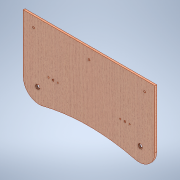
# Autodesk Inventor part: FTC Outside Panels
Saved by Autodesk Inventor 2020 (Build 240168000, 168)
## iProperties
Created: 2022-09-23
Part Number: FTC Outside Panels
Material: Wood (Oak)
Document SubType Name: Modeling
Designer: Jason
Density: 0.76 g/cm^3
Appearance: White Oak - Natural Medium Gloss
Author: Jason
Autodesk Inventor part; units mm, degrees
ref_plane "YZ Plane" through (0, 0, 0) normal (1, 0, 0) x (0, 1, 0)
ref_plane "XZ Plane" through (0, 0, 0) normal (0, 1, 0) x (-1, 0, 0)
ref_plane "XY Plane" through (0, 0, 0) normal (0, 0, 1) x (1, 0, 0)
sketch "Sketch1" plane through (0, 0, 0) normal (0, 0, 1) x (1, 0, 0)
  line L0 (49.2125, 0) -> (54.6328, 0)
  line L1 (357.1875, 0) -> (350.9902, 0)
  arc A0 (0, 49.2125) -> (65.0875, 2.6308) centre (49.2125, 49.2125) ccw
  arc A1 (345.2239, 1.4763) -> (406.4, 49.2125) centre (357.1875, 49.2125) ccw
  arc A2 (203.2, 19.05) -> (54.6328, 0) centre (202.8115, -566.7686) ccw
  arc A3 (350.9902, 0) -> (345.2239, 1.4763) centre (202.8115, -566.7686) ccw
  arc A4 (65.0875, 2.6308) -> (54.6328, 0) centre (202.8115, -566.7686) ccw
  arc A5 (350.9902, 0) -> (203.2, 19.05) centre (202.8115, -566.7686) ccw
  line L2 (0, 49.2125) -> (0, 228.6)
  line L3 (406.4, 228.6) -> (406.4, 49.2125)
  line L4 (0, 228.6) -> (406.4, 228.6)
  point P0 (0, 0)
  point P1 (57.0671, 0.6309)
  constraints: 16 point on circle, 10 end point, 6 centre point, 1 perpendicular, 1 vertical
extrude "Extrusion1" add sketch "Sketch1" along normal blind 5.5563 contours A0 L2 L4 L3 A1 A5 A2
sketch "Sketch2" plane through (0, 0, 5.5563) normal (0, 0, 1) x (1, 0, 0)
  arc A0 (0, 49.2125) -> (57.0671, 0.6309) centre (49.2125, 49.2125) ccw projected
  arc A1 (345.2239, 1.4763) -> (406.4, 49.2125) centre (357.1875, 49.2125) ccw projected
  line L0 (361.7622, 0.2131) -> (361.7412, 44.6631)
  line L1 (361.7412, 44.6631) -> (406.1912, 44.6631)
  line L2 (0.2109, 44.6609) -> (44.6609, 44.6609)
  line L3 (44.6609, 44.6609) -> (44.6609, 0.2109)
  line L4 (365.2681, 38.3131) -> (368.9342, 44.6631)
  line L5 (365.2681, 51.0131) -> (368.9342, 44.6631)
  line L6 (357.9357, 51.0131) -> (365.2681, 51.0131)
  line L7 (357.9357, 38.3131) -> (365.2681, 38.3131)
  line L8 (357.9357, 51.0131) -> (354.2695, 44.6631)
  line L9 (354.2695, 44.6631) -> (357.9357, 38.3131)
  line L10 (48.1878, 38.3109) -> (51.854, 44.6609)
  line L11 (48.1878, 51.0109) -> (51.854, 44.6609)
  line L12 (40.8554, 51.0109) -> (48.1878, 51.0109)
  line L13 (40.8554, 38.3109) -> (48.1878, 38.3109)
  line L14 (40.8554, 51.0109) -> (37.1893, 44.6609)
  line L15 (37.1893, 44.6609) -> (40.8554, 38.3109)
  point P0 (0, 0)
  point P1 (44.6609, 44.6609)
  dimension "d97" = 44.45
  dimension "d99" = 44.45
  dimension "d100" = 44.45
  dimension "d101" = 44.45
  dimension "d102" = 12.7
  dimension "d103" = 12.7
  dimension "d104" = 12.7
  dimension "d105" = 7.3323
  dimension "d106" = 7.3323
  dimension "d107" = 7.3323
  dimension "d108" = 7.3323
  dimension "d109" = 7.3323
  dimension "d110" = 7.3323
  dimension "d111" = 12.7
  dimension "d112" = 12.7
  dimension "d113" = 12.7
  dimension "d114" = 7.3323
  dimension "d115" = 7.3323
  dimension "d116" = 7.3323
  dimension "d117" = 7.3323
  dimension "d118" = 7.3323
  dimension "d119" = 7.3323
  constraints: 32 end point, 6 horizontal, 3 point on circle, 1 perpendicular
  measures "d97" distance of L0.end L0.start
  measures "d99" distance of L0.end L1.end
  measures "d100" distance of L2.start L2.end
  measures "d101" distance of L2.end L3.end
  measures "d102" distance between parallel lines of L5 L9
  measures "d103" distance between parallel lines of L8 L4
  measures "d104" distance between parallel lines of L6 L7
  measures "d105" distance of L8.start L8.end
  measures "d106" distance of L8.end L9.end
  measures "d107" distance of L7.end L4.end
  measures "d108" distance of L9.end L7.end
  measures "d109" distance of L5.start L4.end
  measures "d110" distance of L8.start L6.end
  measures "d111" distance between parallel lines of L11 L15
  measures "d112" distance between parallel lines of L14 L10
  measures "d113" distance between parallel lines of L12 L13
  measures "d114" distance of L14.start L14.end
  measures "d115" distance of L14.end L15.end
  measures "d116" distance of L13.end L10.end
  measures "d117" distance of L15.end L13.end
  measures "d118" distance of L11.start L10.end
  measures "d119" distance of L14.start L12.end
extrude "Extrusion2" cut sketch "Sketch2" against normal blind 5.5563 contours L14 L12 L11 L10 L13 L3 L2 | L2 L3 L13 L15 | L7 L9 L8 L6 L5 L1 L0 | L0 L1 L4 L7
sketch "Sketch3" plane through (0, 0, 5.5563) normal (0, 0, 1) x (1, 0, 0)
  circle A0 centre (92.1534, 86.6412) radius 2.9337
  circle A1 centre (313.9695, 86.6561) radius 2.9337
  line L0 (313.9695, 86.6561) -> (313.9695, 89.539)
  line L1 (313.9695, 86.6561) -> (313.9695, 83.7732)
  line L2 (313.9695, 86.6561) -> (316.4662, 88.0975)
  line L3 (313.9695, 86.6561) -> (311.4729, 88.0975)
  line L4 (313.9695, 86.6561) -> (311.4729, 85.2146)
  line L5 (313.9695, 86.6561) -> (316.4662, 85.2146)
  line L6 (316.4662, 88.0975) -> (316.4662, 85.2146)
  line L7 (316.4662, 88.0975) -> (313.9695, 89.539)
  line L8 (311.4729, 88.0975) -> (313.9695, 89.539)
  line L9 (311.4729, 88.0975) -> (311.4729, 85.2146)
  line L10 (311.4729, 85.2146) -> (313.9695, 83.7732)
  line L11 (313.9695, 83.7732) -> (316.4662, 85.2146)
  line L12 (92.1534, 86.6546) -> (92.1534, 89.5375)
  line L13 (92.1534, 86.6546) -> (92.1534, 83.7717)
  line L14 (92.1534, 86.6546) -> (94.65, 88.096)
  line L15 (92.1534, 86.6546) -> (89.6567, 88.096)
  line L16 (92.1534, 86.6546) -> (89.6567, 85.2131)
  line L17 (92.1534, 86.6546) -> (94.65, 85.2131)
  line L18 (94.65, 88.096) -> (94.65, 85.2131)
  line L19 (94.65, 88.096) -> (92.1534, 89.5375)
  line L20 (89.6567, 88.096) -> (92.1534, 89.5375)
  line L21 (89.6567, 88.096) -> (89.6567, 85.2131)
  line L22 (89.6567, 85.2131) -> (92.1534, 83.7717)
  line L23 (92.1534, 83.7717) -> (94.65, 85.2131)
  line L24 (40.8554, 51.0109) -> (48.2089, 38.2743)
  line L25 (40.8554, 51.0109) -> (37.1893, 44.6609) projected
  line L26 (51.854, 44.6609) -> (48.1878, 51.0109) projected
  line L27 (37.1893, 44.6609) -> (51.854, 44.6609)
  line L28 (48.1878, 51.0109) -> (40.8554, 51.0109) projected
  line L29 (40.8554, 38.3109) -> (48.1878, 51.0109)
  line L30 (365.2681, 38.3131) -> (368.9342, 44.6631) projected
  line L31 (357.9357, 51.0131) -> (365.2681, 38.3131)
  line L32 (354.2695, 44.6631) -> (368.9342, 44.6631)
  line L33 (365.2681, 51.0131) -> (357.9357, 51.0131) projected
  line L34 (357.9357, 38.3131) -> (365.2681, 38.3131) projected
  line L35 (365.2681, 51.0131) -> (357.9357, 38.3131)
  line L36 (44.5216, 44.6609) -> (361.6019, 44.6631)
  line L37 (44.5216, 44.6609) -> (92.1534, 86.6546)
  line L38 (361.6019, 44.6631) -> (313.9695, 86.6561)
  point P0 (0, 0)
  dimension "d20" = 5.8674
  dimension "d23" = 5.8674
  dimension "d58" = 2.8829
  dimension "d59" = 2.8829
  dimension "d60" = 2.8829
  dimension "d61" = 60
  dimension "d62" = 2.8829
  dimension "d63" = 2.8829
  dimension "d64" = 60
  dimension "d65" = 60
  dimension "d66" = 2.8829
  dimension "d67" = 60
  dimension "d69" = 2.8829
  dimension "d70" = 2.8829
  dimension "d71" = 2.8829
  dimension "d72" = 60
  dimension "d73" = 2.8829
  dimension "d74" = 2.8829
  dimension "d75" = 60
  dimension "d76" = 60
  dimension "d77" = 2.8829
  dimension "d78" = 60
  dimension "d126" = 63.5
  dimension "d127" = 41.4
  dimension "d128" = 63.5
  dimension "d129" = 41.4
  constraints: 66 end point, 4 vertical, 2 centre point, 2 horizontal, 2 midpoint
  measures "d20" diameter of A0
  measures "d23" diameter of A1
  measures "d58" distance of L0.start L0.end
  measures "d59" distance of L0.start L1.end
  measures "d60" distance of L0.start L2.end
  measures "d61" angle of L2 L0
  measures "d62" distance of L0.start L3.end
  measures "d63" distance of L0.start L4.end
  measures "d64" angle of L3 L0
  measures "d65" angle of L4 L3
  measures "d66" distance of L0.start L5.end
  measures "d67" angle of L5 L2
  measures "d69" distance of L14.start L19.end
  measures "d70" distance of L14.start L22.end
  measures "d71" distance of L14.start L14.end
  measures "d72" angle of L14 L12
  measures "d73" distance of L14.start L15.end
  measures "d74" distance of L14.start L16.end
  measures "d75" angle of L15 L12
  measures "d76" angle of L16 L15
  measures "d77" distance of L14.start L17.end
  measures "d78" angle of L17 L14
  measures "d126" distance of L36.start L37.end
  measures "d127" angle of L36 L37
  measures "d128" distance of L36.end L38.end
  measures "d129" angle of L36 L38
extrude "Extrusion4" cut sketch "Sketch3" against normal blind 5.5563 contours L3 L8 L0 | L38 L11 L1 | L0 L7 L2 | L4 L9 L3 | L1 L10 L4 | L2 L6 L5 | L5 L11 L38 | L15 L20 L12 | L17 L23 L13 | L12 L19 L14 | L16 L21 L15 | L37 L22 L16 | L14 L18 L17 | L13 L22 L37
sketch "Sketch4" plane through (0, 0, 5.5563) normal (0, 0, 1) x (1, 0, 0)
  line L0 (91.8966, 105.3714) -> (91.8966, 105.3714)
  line L1 (92.1466, 105.4384) -> (108.4072, 96.049)
  line L2 (92.1466, 67.8861) -> (108.4072, 77.2742)
  circle A0 centre (92.1466, 102.6622) radius 2
  circle A1 centre (106.003, 78.6622) radius 2
  circle A2 centre (106.003, 94.6622) radius 2
  line L3 (108.4072, 77.2742) -> (108.4072, 96.049)
  line L4 (75.886, 77.2742) -> (75.886, 96.049)
  line L5 (92.1466, 105.4384) -> (75.886, 96.049)
  circle A3 centre (78.2902, 94.6622) radius 2
  circle A4 centre (92.1466, 70.6622) radius 2
  circle A5 centre (78.2902, 78.6622) radius 2
  line L6 (92.1466, 67.8861) -> (75.886, 77.2742)
  circle A6 centre (92.1466, 86.6622) radius 6.35
  circle A7 centre (99.239, 74.3758) radius 1.8542
  circle A8 centre (106.337, 86.6619) radius 1.905
  circle A9 centre (99.2318, 98.9527) radius 1.8542
  circle A10 centre (85.0637, 98.9527) radius 1.8542
  circle A11 centre (85.0637, 74.3758) radius 1.8542
  circle A12 centre (77.96, 86.6632) radius 1.905
  circle A13 centre (327.8333, 94.6644) radius 2
  line L7 (330.2375, 77.2763) -> (330.2375, 96.0512)
  circle A14 centre (327.8333, 78.6644) radius 2
  circle A15 centre (328.1673, 86.6641) radius 1.905
  circle A16 centre (321.0693, 74.3779) radius 1.8542
  line L8 (313.9769, 67.8882) -> (330.2375, 77.2763)
  circle A17 centre (313.9769, 70.6644) radius 2
  circle A18 centre (306.894, 74.3779) radius 1.8542
  circle A19 centre (300.1205, 78.6644) radius 2
  line L9 (313.9769, 67.8882) -> (297.7162, 77.2763)
  line L10 (313.9769, 105.4406) -> (330.2375, 96.0512)
  circle A20 centre (321.0621, 98.9548) radius 1.8542
  circle A21 centre (313.9769, 86.6644) radius 6.35
  circle A22 centre (313.9769, 102.6644) radius 2
  line L11 (297.7162, 77.2763) -> (297.7162, 96.0512)
  circle A23 centre (299.7903, 86.6654) radius 1.905
  circle A24 centre (306.894, 98.9548) radius 1.8542
  circle A25 centre (300.1205, 94.6644) radius 2
  line L12 (313.9769, 105.4406) -> (297.7162, 96.0512)
  line L13 (313.7269, 105.3736) -> (313.7269, 105.3736)
  line L14 (40.8554, 38.3109) -> (37.1893, 44.6609) projected
  line L15 (37.1893, 44.6609) -> (51.854, 44.6609)
  line L16 (51.854, 44.6609) -> (135.3148, 44.6609)
  line L17 (44.5216, 44.6609) -> (44.5216, 125.7986)
  line L18 (368.9342, 44.6631) -> (365.2681, 38.3131) projected
  line L19 (368.9342, 44.6631) -> (291.9527, 44.6631)
  line L20 (361.6019, 44.6631) -> (361.6019, 118.2501)
  point P0 (0, 0)
  point P1 (92.1534, 89.5375)
  dimension "d81" = 12.7
  dimension "d82" = 3.81
  dimension "d83" = 3.81
  dimension "d84" = 3.7084
  dimension "d85" = 3.7084
  dimension "d86" = 3.7084
  dimension "d87" = 3.7084
  dimension "d88" = 12.7
  dimension "d89" = 3.81
  dimension "d90" = 3.81
  dimension "d91" = 3.7084
  dimension "d92" = 3.7084
  dimension "d93" = 3.7084
  dimension "d94" = 3.7084
  dimension "d120" = 63.5
  dimension "d121" = 47.625
  dimension "d122" = 42.0013
  dimension "d123" = 63.5
  dimension "d124" = 47.625
  dimension "d125" = 42.0013
  constraints: 38 end point, 26 centre point, 2 horizontal, 2 point on line, 2 vertical, 1 midpoint
  measures "d81" diameter of A6
  measures "d82" diameter of A8
  measures "d83" diameter of A12
  measures "d84" diameter of A10
  measures "d85" diameter of A9
  measures "d86" diameter of A7
  measures "d87" diameter of A11
  measures "d88" diameter of A21
  measures "d89" diameter of A15
  measures "d90" diameter of A23
  measures "d91" diameter of A24
  measures "d92" diameter of A20
  measures "d93" diameter of A16
  measures "d94" diameter of A18
  measures "d120" distance of L17.start point (92.147, 86.662)
  measures "d121" distance from line of L17 point (92.147, 86.662)
  measures "d122" distance from line of L16 point (92.147, 86.662)
  measures "d123" distance of L20.start point (313.977, 86.664)
  measures "d124" distance from line of L20 point (313.977, 86.664)
  measures "d125" distance from line of L19 point (313.977, 86.664)
extrude "Extrusion5" cut sketch "Sketch4" against normal blind 5.5626 contours A8 | A12 | A15 | A23
sketch "Sketch5" plane through (-0.198, 12.7962, 5.5563) normal (0, 0, 1) x (1, 0, 0)
  circle A0 centre (31.948, 184.0538) radius 2.9337
  circle A1 centre (374.848, 184.0538) radius 2.9337
  line L0 (31.948, 184.0538) -> (203.398, 184.0538)
  circle A2 centre (203.398, 184.0538) radius 2.9337
  point P0 (0.198, 215.8038)
  dimension "d141" = 5.8674
  dimension "d140" = 5.8674
  dimension "d139" = 171.45
  dimension "d138" = 5.8674
  constraints: 3 centre point, 2 end point, 1 coincident, 1 horizontal
  measures "d141" diameter of A0
  measures "d140" diameter of A1
  measures "d139" distance of L0.start L0.end
  measures "d138" diameter of A2
extrude "Extrusion6" cut sketch "Sketch5" against normal up to surface (5.5563 mm away)
body "Solid1"
